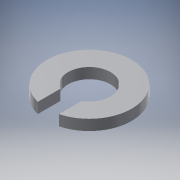
# Autodesk Inventor part: Retaining Ring
Saved by Autodesk Inventor 2019 (Build 230136000, 136)
## iProperties
Created: 2013-01-30
Part Number: Retaining Ring
Material: Aluminum 6061
Document SubType Name: Modeling
Designer: banachd
Density: 1 g/cm^3
Description: 2 mm RETAINING RING
Appearance: Aluminum - Flat
Author: banachd
Autodesk Inventor part; units mm, degrees
ref_plane "YZ Plane" through (0, 0, 0) normal (1, 0, 0) x (0, 1, 0)
ref_plane "XZ Plane" through (0, 0, 0) normal (0, 1, 0) x (-1, 0, 0)
ref_plane "XY Plane" through (0, 0, 0) normal (0, 0, 1) x (1, 0, 0)
sketch "Sketch1" plane through (0, 0, 0) normal (0, 0, 1) x (1, 0, 0)
  arc A0 (0.5, -0.866) -> (-0.5, -0.866) centre (0, 0) ccw
  arc A1 (0.5, -1.9365) -> (-0.5, -1.9365) centre (0, 0) ccw
  line L0 (-0.5, -0.866) -> (-0.5, -1.9365)
  line L1 (0.5, -0.866) -> (0.5, -1.9365)
  dimension "d0" = 2
  dimension "d1" = 4
  dimension "d28" = 1
  constraints: 4 end point, 4 point on circle, 2 centre point, 2 coincident, 2 vertical, 1 horizontal alignment
  measures "d0" diameter of A0
  measures "d1" diameter of A1
  measures "d28" distance of L1.end L0.end
extrude "Extrusion1" add sketch "Sketch1" along normal blind 0.5
equation "\"d13\" = 18.5"
equation "\"d14\" = 4.45"
equation "\"d15\" = 0.67"
equation "\"d16\" = 2"
equation "\"d17\" = 2.68"
equation "\"d18\" = 8.5"
equation "\"d19\" = 11.2"
equation "\"d20\" = 2.5"
equation "\"d21\" = 4.5"
equation "\"d22\" = 14.5"
body "Solid1"
